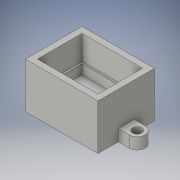
# Autodesk Inventor part: fc-GyroAccelBoxTop
Saved by Autodesk Inventor 2016 SP1 (Build 200210100, 210)
## iProperties
Created: 2016-02-16
Part Number: fc-GyroAccelBoxTop
Material: Generic
Document SubType Name: Modeling
Designer: Faith
Density: 1 g/cm^3
Appearance: Default
Author: Faith
Autodesk Inventor part; units mm, degrees
ref_plane "YZ Plane" through (0, 0, 0) normal (1, 0, 0) x (0, 1, 0)
ref_plane "XZ Plane" through (0, 0, 0) normal (0, 1, 0) x (-1, 0, 0)
ref_plane "XY Plane" through (0, 0, 0) normal (0, 0, 1) x (1, 0, 0)
sketch "Sketch1" plane through (0, 0, 0) normal (0, 1, 0) x (-1, 0, 0)
  line L0 (20.193, 15.748) -> (-20.193, 15.748)
  line L1 (-20.193, -15.748) -> (20.193, -15.748)
  line L2 (20.193, 15.748) -> (-20.193, -15.748) construction
  line L3 (-20.193, 15.748) -> (20.193, -15.748) construction
  line L4 (26.2784, 0) -> (13.1572, 0) construction
  line L5 (26.2784, 4.445) -> (20.193, 4.445)
  line L6 (20.193, -4.445) -> (26.2784, -4.445)
  arc A0 (26.2784, -4.445) -> (26.2784, 4.445) centre (26.2784, 0) ccw
  line L7 (0, -15.748) -> (0, 15.748) construction
  line L8 (-26.2784, 4.445) -> (-20.193, 4.445)
  line L9 (-20.193, -4.445) -> (-26.2784, -4.445)
  arc A1 (-26.2784, 4.445) -> (-26.2784, -4.445) centre (-26.2784, 0) ccw
  line L10 (20.193, -15.748) -> (20.193, -4.445)
  line L11 (20.193, 4.445) -> (20.193, 15.748)
  line L12 (-20.193, 15.748) -> (-20.193, 4.445)
  line L13 (-20.193, -4.445) -> (-20.193, -15.748)
  circle A2 centre (-26.2784, 0) radius 2.5527
  circle A3 centre (26.2784, 0) radius 2.5527
  point P0 (0, 0)
  point P1 (19.7178, 0)
  dimension "d0" = 40.386
  dimension "d1" = 31.496
  dimension "d2" = 8.89
  dimension "d5" = 5.1054
  dimension "d6" = 5.1054
  constraints: 30 end point, 7 parallel, 5 midpoint, 5 symmetric about line, 4 centre point, 4 coincident, 4 point on circle, 2 horizontal, 2 perpendicular, 2 tangent, 1 collinear, 1 other
  measures "d0" distance of L1.start L1.end
  measures "d1" distance of L0.end L1.start
  measures "d2" distance between parallel lines of L6 L5
  measures "d5" diameter of A2
  measures "d6" diameter of A3
extrude "Extrusion2" add sketch "Sketch1" along normal blind 6.35
sketch "Sketch2" plane through (0, 6.35, 0) normal (0, 1, 0) x (1, 0, 0)
  line L0 (20.193, 15.748) -> (-20.193, 15.748) projected
  line L1 (-20.193, 15.748) -> (20.193, 15.748)
  line L2 (20.193, 15.748) -> (20.193, -15.748)
  line L3 (20.193, -15.748) -> (-20.193, -15.748)
  line L4 (-20.193, -15.748) -> (-20.193, 15.748)
  line L5 (-16.891, -12.446) -> (16.891, -12.446)
  line L6 (16.891, -12.446) -> (16.891, 12.446)
  line L7 (16.891, 12.446) -> (-16.891, 12.446)
  line L8 (-16.891, 12.446) -> (-16.891, -12.446)
  line L9 (-16.891, -12.446) -> (16.891, 12.446) construction
  line L10 (16.891, -12.446) -> (-16.891, 12.446) construction
  point P0 (0, 0)
  dimension "d9" = 3.302
  dimension "d10" = 3.302
  constraints: 20 end point, 4 parallel, 2 horizontal, 2 midpoint, 2 perpendicular
  measures "d9" distance between parallel lines of L4 L8
  measures "d10" distance between parallel lines of L0 L7
extrude "Extrusion3" add sketch "Sketch2" along normal blind 19.05
sketch "Sketch3" plane through (0, 6.35, 0) normal (0, 1, 0) x (1, 0, 0)
  line L0 (-16.891, 12.446) -> (-16.891, -12.446) projected
  line L1 (-16.891, -12.446) -> (16.891, -12.446) projected
  line L2 (16.891, 12.446) -> (-16.891, 12.446) projected
  line L3 (-16.891, 12.446) -> (16.891, 12.446)
  line L4 (16.891, 12.446) -> (16.891, -12.446)
  line L5 (16.891, -12.446) -> (-16.891, -12.446)
  line L6 (-16.891, -12.446) -> (-16.891, 12.446)
  line L7 (-15.875, -11.43) -> (15.875, -11.43)
  line L8 (15.875, -11.43) -> (15.875, 11.43)
  line L9 (15.875, 11.43) -> (-15.875, 11.43)
  line L10 (-15.875, 11.43) -> (-15.875, -11.43)
  line L11 (-15.875, -11.43) -> (15.875, 11.43) construction
  line L12 (15.875, -11.43) -> (-15.875, 11.43) construction
  point P0 (0, 0)
  dimension "d13" = 1.016
  dimension "d14" = 1.016
  constraints: 20 end point, 4 parallel, 2 horizontal, 2 midpoint, 2 perpendicular
  measures "d13" distance between parallel lines of L2 L9
  measures "d14" distance between parallel lines of L0 L10
extrude "Extrusion4" add sketch "Sketch3" along normal blind 5.334
equation "\"d0\" = 2 * imuBoxWallThickness + imuBoardLength + 2 * imuPrintError"
equation "\"d1\" = 2 * imuBoxWallThickness + imuBoardWidth + 2 * imuPrintError"
equation "\"d2\" = widthSlot"
equation "\"d7\" = imuBoxBottom"
equation "\"d9\" = imuBoxWallThickness - imuPrintError"
equation "\"d10\" = imuBoxWallThickness - imuPrintError"
equation "\"d11\" = imuBoxHeight"
equation "\"d15\" = imuBoardBottomThickness"
equation "\"imuBoardWidth\" = 22.86"
equation "\"imuBoardLength\" = 31.75"
equation "\"imuBoardTopThickness\" = 11.176"
equation "\"imuBoardBottomThickness\" = 5.334"
equation "\"imuBoardHoleDistance\" = 19.7104"
equation "\"imuBoxWallThickness\" = 3.81"
equation "\"widthSlot\" = 8.89"
equation "\"imuBoxBottom\" = 6.35"
equation "\"imuBoxHeight\" = 19.05"
equation "\"imuPrintError\" = 0.508"
body "Solid2"
